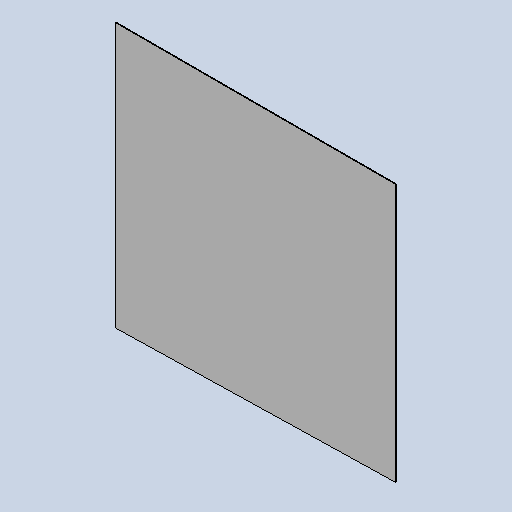
# Autodesk Inventor part: GBK 2111 shield 1
Saved by Autodesk Inventor 2026.2 (Build 302298010, 298A)
## iProperties
Created: 2026-04-17
Part Number: GBK 2111 shield 1
Material: Steel
Document SubType Name: Sheet Metal
Designer: pokla
Stock Number: 2111
Mass: 64141 g
Surface Area: 41083 cm^2
Volume: 8170.83 cm^3
Density: 7.85 g/cm^3
Sheet Metal Rule: Default_mm
Sheet Metal Width: 1396,640 mm
Sheet Metal Length: 1511,313 mm
Sheet Metal Area: 2110761,204 mm^2
Appearance: Default
Flat Pattern Width: 139.664 cm
Flat Pattern Length: 151.131 cm
Flat Pattern Area: 21107.6 cm^2
Author: admin
Autodesk Inventor part; units mm, degrees
ref_plane "YZ Plane" through (0, 0, 0) normal (1, 0, 0) x (0, 1, 0)
ref_plane "XZ Plane" through (0, 0, 0) normal (0, 1, 0) x (-1, 0, 0)
ref_plane "XY Plane" through (0, 0, 0) normal (0, 0, 1) x (1, 0, 0)
sketch "Sketch1" plane through (0, 0, 0) normal (0, 0, 1) x (1, 0, 0)
  line L0 (740, -745) -> (-740, -745)
  line L1 (-740, -745) -> (-740, 745)
  line L2 (-740, 745) -> (740, 745)
  line L3 (740, 745) -> (740, -745)
  line L4 (740, -745) -> (-740, 745) construction
  line L5 (-740, -745) -> (740, 745) construction
  line L6 (-740, -652) -> (740, -618.4141)
  point P0 (0, 0)
  dimension "d0" = 1480
  dimension "d1" = 1490
  dimension "d3" = 1.3
  dimension "d4" = 93
  measures "d0" distance of L1.end L2.end
  measures "d1" distance of L0.end L1.end
  measures "d3" angle of L0 L6
  measures "d4" distance of L0.end L6.start
extrude "Plate1" add sketch "Sketch1" along normal blind 4 contours L6 L1 L2 L3
sketch "Sketch3" plane through (0, 0, 0) normal (0, 0, -1) x (-1, 0, 0)
  line L0 (562.4602, -535.2203) -> (562.4602, -892.9108) construction
  line L1 (562.4602, -892.9108) -> (533.3905, -892.9108) construction
  line L2 (533.3905, -892.9108) -> (533.3905, -535.2203) construction
  line L3 (533.3905, -535.2203) -> (562.4602, -535.2203) construction
  line L4 (710, -491) -> (770, -491) projected
  line L5 (710, -491) -> (710, -487) projected
  line L6 (669.8628, -494.5) -> (669.8628, -591.5) projected
  line L7 (669.8628, -591.5) -> (665.8638, -591.5) projected
  line L8 (710, 5.6667) -> (770, 5.6667) projected
  line L9 (710, 5.6667) -> (710, 9.6667) projected
  line L10 (710, 502.3333) -> (770, 502.3333) projected
  line L11 (710, 502.3333) -> (710, 506.3333) projected
  ellipse E0 centre (669.8628, 743.5) end of major axis (669.8628, 773.5) minor radius 0.6803 (669.8628, 713.5) -> (669.8628, 773.5) ccw projected
  line L12 (669.8628, 713.5) -> (665.8638, 713.5) projected
  ellipse E1 centre (169.7342, 743.5) end of major axis (169.7342, 773.5) minor radius 0.6803 (169.7342, 713.5) -> (169.7342, 773.5) ccw projected
  line L13 (169.7342, 713.5) -> (165.7352, 713.5) projected
  ellipse E2 centre (-330.3944, 743.5) end of major axis (-330.3944, 773.5) minor radius 0.6803 (-330.3944, 713.5) -> (-330.3944, 773.5) ccw projected
  line L14 (-330.3944, 713.5) -> (-334.3934, 713.5) projected
  line L15 (-738.6395, 502.3333) -> (-680, 502.3333) projected
  line L16 (-680, 502.3333) -> (-680, 506.3333) projected
  line L17 (-738.6395, 5.6667) -> (-680, 5.6667) projected
  line L18 (-680, 5.6667) -> (-680, 9.6667) projected
  line L19 (-738.6395, -491) -> (-680, -491) projected
  line L20 (-680, -491) -> (-680, -487) projected
  line L21 (-330.3944, -494.5) -> (-330.3944, -591.5) projected
  line L22 (-330.3944, -591.5) -> (-334.3934, -591.5) projected
  line L23 (169.7342, -494.5) -> (169.7342, -591.5) projected
  line L24 (169.7342, -591.5) -> (165.7352, -591.5) projected
  point P0 (0, 0)
  constraints: 5 other
mark "Mark2"
equation "\"d0\" = Лист_ширина"
equation "\"d1\" = 0.5 * Лист_длина"
equation "\"d2\" = Thickness"
equation "\"BendRadius\" = Thickness"
equation "\"BendReliefWidth\" = Thickness"
equation "\"BendReliefDepth\" = 0.5 * Thickness"
equation "\"CornerReliefSize\" = 4 * Thickness"
equation "\"MinimumRemnant\" = 2 * Thickness"
equation "\"TransitionRadius\" = BendRadius"
equation "\"JacobiRadiusSize\" = BendRadius"
equation "\"GapSize\" = Thickness"
equation "\"Лист_ширина\" = 1480"
equation "\"Лист_длина\" = 2980"
equation "\"Thickness\" = 4"
body "Solid1"
